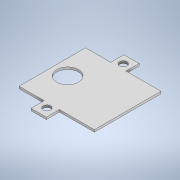
# Autodesk Inventor part: lid 4.0
Saved by Autodesk Inventor 2020.2 (Build 242310000, 310)
## iProperties
Created: 2020-02-13
Part Number: lid 4.0
Material: Generic
Document SubType Name: Modeling
Designer: ColinP
Density: 1 g/cm^3
Appearance: Default
Author: ColinP
Autodesk Inventor part; units mm, degrees
ref_plane "YZ Plane" through (0, 0, 0) normal (1, 0, 0) x (0, 1, 0)
ref_plane "XZ Plane" through (0, 0, 0) normal (0, 1, 0) x (-1, 0, 0)
ref_plane "XY Plane" through (0, 0, 0) normal (0, 0, 1) x (1, 0, 0)
sketch "Sketch1" plane through (0, 0, 0) normal (0, 1, 0) x (-1, 0, 0)
  line L0 (8.0078, 6.9217) -> (-26.4922, 6.9217)
  line L1 (-26.4922, 6.9217) -> (-26.4922, -23.5583)
  line L2 (-26.4922, -23.5583) -> (8.0078, -23.5583)
  line L3 (8.0078, -23.5583) -> (8.0078, 6.9217)
  point P0 (0, 0)
  dimension "d0" = 34.5
  dimension "d1" = 30.48
  constraints: 8 end point, 2 parallel, 1 horizontal, 1 perpendicular
  measures "d0" distance of L2.end L1.end
  measures "d1" distance of L1.end L0.end
extrude "Extrusion1" add sketch "Sketch1" along normal blind 1
sketch "Sketch2" plane through (0, 1, 0) normal (0, 1, 0) x (1, 0, 0)
  line L0 (-8.0078, 23.5583) -> (-8.0078, -6.9217) projected
  line L1 (-8.0078, -6.9217) -> (-8.0078, -5.9217)
  line L2 (-8.0078, -5.9217) -> (-7.0078, -5.9217)
  line L3 (26.4922, -6.9217) -> (26.4922, 23.5583) projected
  line L4 (26.4922, 23.5583) -> (26.4922, 22.5583)
  line L5 (26.4922, 22.5583) -> (25.4922, 22.5583)
  line L6 (-7.0078, -5.9217) -> (25.4922, -5.9217)
  line L7 (25.4922, -5.9217) -> (25.4922, 22.5583)
  line L8 (25.4922, 22.5583) -> (-7.0078, 22.5583)
  line L9 (-7.0078, 22.5583) -> (-7.0078, -5.9217)
  line L10 (-8.0078, 23.5583) -> (-8.0078, -6.9217) projected
  line L11 (-8.0078, -6.9217) -> (26.4922, -6.9217) projected
  line L12 (26.4922, -6.9217) -> (26.4922, 23.5583) projected
  line L13 (26.4922, 23.5583) -> (-8.0078, 23.5583) projected
  point P0 (0, 0)
  dimension "d4" = 1
  dimension "d5" = 1
  dimension "d6" = 1
  dimension "d7" = 1
  constraints: 16 end point, 3 perpendicular, 2 parallel, 2 point on line, 1 horizontal
  measures "d4" distance of L0.end L1.end
  measures "d5" distance of L1.end L2.end
  measures "d6" distance of L3.end L4.end
  measures "d7" distance of L4.end L5.end
extrude "Extrusion2" add sketch "Sketch2" along normal blind 2 contours L13 L3 L5 L8 L9 L2 L0 | L2 L6 L7 L5 L3 L11 L0
sketch "Sketch3" plane through (0, 0, 0) normal (0, 1, 0) x (1, 0, 0)
  line L0 (-7.0078, -5.9217) -> (-7.0078, 22.5583) projected
  line L1 (-7.0078, 8.3183) -> (6.9922, 8.3183)
  line L2 (6.9922, 8.3183) -> (6.9922, 25.8183)
  line L3 (6.9922, 25.8183) -> (6.9922, -9.1817)
  circle A0 centre (6.9922, -9.1817) radius 1.7
  circle A1 centre (6.9922, 25.8183) radius 1.7
  line L4 (25.4922, -5.9217) -> (-7.0078, -5.9217) projected
  line L5 (6.9922, -5.9217) -> (3.4922, -5.9217)
  line L6 (3.4922, -5.9217) -> (3.4922, -12.9217)
  line L7 (3.4922, -12.9217) -> (10.4922, -12.9217)
  line L8 (10.4922, -12.9217) -> (10.4922, -5.9217)
  line L9 (-7.0078, 22.5583) -> (25.4922, 22.5583) projected
  line L10 (3.4922, 22.5583) -> (3.4922, 29.5583)
  line L11 (3.4922, 29.5583) -> (10.4922, 29.5583)
  line L12 (10.4922, 29.5583) -> (10.4922, 22.5583)
  point P0 (0, 0)
  point P1 (9.2422, 22.5583)
  dimension "d10" = 14
  dimension "d11" = 17.5
  dimension "d12" = 35
  dimension "d13" = 3.4
  dimension "d14" = 3.4
  dimension "d15" = 3.5
  dimension "d16" = 7
  dimension "d17" = 7
  dimension "d18" = 7
  dimension "d31" = 7
  constraints: 20 end point, 9 point on line, 5 perpendicular, 2 centre point, 2 coincident, 2 midpoint, 1 horizontal, 1 vertical
  measures "d10" distance of L1.start L1.end
  measures "d11" distance of L1.end L2.end
  measures "d12" distance of L2.end L3.end
  measures "d13" diameter of A0
  measures "d14" diameter of A1
  measures "d15" distance of L5.start L5.end
  measures "d16" distance of L5.end L6.end
  measures "d17" distance of L6.end L7.end
  measures "d18" distance of L10.start L10.end
  measures "d31" distance of L10.end L11.end
extrude "Extrusion3" add sketch "Sketch3" along normal blind 1 contours L4 L8 L7 L6 | L10 L11 L12 L9
sketch "Sketch4" plane through (0, 1, 0) normal (0, 1, 0) x (1, 0, 0)
  line L0 (-7.0078, -5.9217) -> (-7.0078, 22.5583) projected
  line L1 (-7.0078, 8.3183) -> (-1.0078, 8.3183)
  point P0 (0, 0)
  dimension "d21" = 6
  constraints: 2 end point, 1 horizontal, 1 midpoint
  measures "d21" distance of L1.start L1.end
hole "Hole1" at (-1.0078, 1, -8.3183) direction (0, -1, 0) diameter 10 end through all
sketch "Sketch5" plane through (0, 3, 0) normal (0, 1, 0) x (1, 0, 0)
  line L0 (26.4922, 23.5583) -> (-8.0078, 23.5583) projected
  line L1 (-8.0078, 23.5583) -> (-8.0078, -6.9217) projected
  line L2 (-8.0078, -6.9217) -> (26.4922, -6.9217) projected
  line L3 (26.4922, -6.9217) -> (26.4922, 23.5583) projected
  line L4 (-7.0078, 22.5583) -> (25.4922, 22.5583) projected
  line L5 (25.4922, 22.5583) -> (25.4922, -5.9217) projected
  line L6 (25.4922, -5.9217) -> (-7.0078, -5.9217) projected
  line L7 (-7.0078, -5.9217) -> (-7.0078, 22.5583) projected
  point P0 (0, 0)
extrude "Extrusion4" cut sketch "Sketch5" against normal blind 2
body "Solid1"
